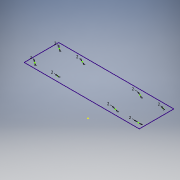
# Autodesk Inventor part: APOIO_PERFIL_STRUTURAL
Saved by Autodesk Inventor 2018 (Build 220112000, 112)
## iProperties
Created: 2018-10-09
Part Number: APOIO_PERFIL_STRUTURAL
Material: Genérico
Document SubType Name: Modeling
Designer: Georgines
Density: 1 g/cm^3
Appearance: Padrão
Author: Georgines
Autodesk Inventor part; units mm, degrees
ref_plane "YZ Plane" through (0, 0, 0) normal (1, 0, 0) x (0, 1, 0)
ref_plane "XZ Plane" through (0, 0, 0) normal (0, 1, 0) x (-1, 0, 0)
ref_plane "XY Plane" through (0, 0, 0) normal (0, 0, 1) x (1, 0, 0)
sketch "Esboço1" plane through (0, 0, 0) normal (0, 0, 1) x (1, 0, 0)
  line L0 (45, 21.6235) -> (-105, 21.6235)
  line L1 (-105, 21.6235) -> (-105, 66.6235)
  line L2 (-105, 66.6235) -> (45, 66.6235)
  line L3 (45, 66.6235) -> (45, 21.6235)
  circle A0 centre (37.5, 28.1235) radius 1 construction
  circle A1 centre (7.5, 28.1235) radius 1 construction
  circle A2 centre (-67.5, 28.1235) radius 1 construction
  circle A3 centre (-97.5, 28.1235) radius 1 construction
  circle A4 centre (-97.5, 60.1235) radius 1 construction
  circle A5 centre (-67.5, 60.1235) radius 1 construction
  circle A6 centre (7.5, 60.1235) radius 1 construction
  circle A7 centre (37.5, 60.1235) radius 1 construction
  line L4 (45, 21.6235) -> (45, -58.3765) construction
  line L5 (45, -58.3765) -> (5, -58.3765) construction
  line L6 (5, -58.3765) -> (-105, 21.6235) construction
  point P0 (0, 0)
  dimension "d0" = 2
  dimension "d1" = 2
  dimension "d2" = 2
  dimension "d3" = 2
  dimension "d4" = 2
  dimension "d5" = 2
  dimension "d6" = 2
  dimension "d7" = 2
  dimension "d8" = 80
  dimension "d9" = 40
  constraints: 14 end point, 8 centre point, 2 parallel, 2 perpendicular, 1 horizontal, 1 vertical
  measures "d0" diameter of A0
  measures "d1" diameter of A1
  measures "d2" diameter of A2
  measures "d3" diameter of A3
  measures "d4" diameter of A4
  measures "d5" diameter of A5
  measures "d6" diameter of A6
  measures "d7" diameter of A7
  measures "d8" distance of L0.start L4.end
  measures "d9" distance of L4.end L5.end
extrude "Extrusão1" add sketch "Esboço1" along normal blind 9.52
